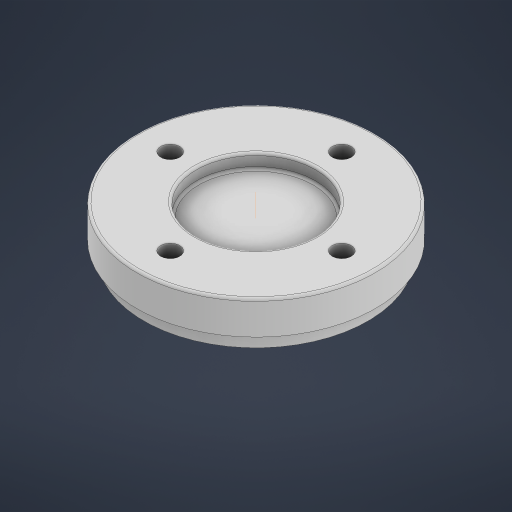
# Autodesk Inventor part: sf_Cylinder_Front_Lid_1
Saved by Autodesk Inventor 2024 (Build 280153000, 153)
## iProperties
Created: 2024-03-20
Part Number: sf_Cylinder_Front_Lid_1
Material: Generisch
Document SubType Name: Modeling
Designer: Simon
Density: 1 g/cm^3
Appearance: Vorgabe
Author: Simon
Autodesk Inventor part; units mm, degrees
ref_plane "YZ Plane" through (0, 0, 0) normal (1, 0, 0) x (0, 1, 0)
ref_plane "XZ Plane" through (0, 0, 0) normal (0, 1, 0) x (-1, 0, 0)
ref_plane "XY Plane" through (0, 0, 0) normal (0, 0, 1) x (1, 0, 0)
sketch "Skizze1" plane through (0, 0, 0) normal (1, 0, 0) x (0, 1, 0)
  line L0 (12.5, 3) -> (12.5, -3) construction
  line L1 (-12.5, -3) -> (-12.5, 3) construction
  line L2 (6, 26.2642) -> (6, -26.2642) construction
  line L3 (-6, -26.2642) -> (-6, 26.2642) construction
  line L4 (14, 26.2642) -> (14, -26.2642) construction
  line L5 (-14, -26.2642) -> (-14, 26.2642) construction
  line L6 (23.5, 26.2642) -> (23.5, -26.2642) construction
  line L7 (-23.5, -26.2642) -> (-23.5, 26.2642) construction
  line L8 (12.5, -3) -> (0, -3)
  line L9 (0, -3) -> (0, -8)
  line L10 (0, -8) -> (6, -8)
  line L11 (6, -8) -> (6, -13)
  line L12 (6, -13) -> (14, -13)
  line L13 (14, -13) -> (14, -10)
  line L14 (25, 26.2642) -> (25, -26.2642) construction
  line L15 (-25, -26.2642) -> (-25, 26.2642) construction
  line L16 (14, -10) -> (23.5, -10)
  line L17 (23.5, -10) -> (23.5, -7)
  line L18 (23.5, -7) -> (25, -7)
  line L19 (25, -7) -> (25, 0)
  line L20 (12.5, -3) -> (12.5, 0)
  line L21 (25, 0) -> (12.5, 0)
  point P0 (0, 0)
  dimension "d1" = 6
  dimension "d5" = 5
  dimension "d6" = 6
  dimension "d7" = 5
  dimension "d8" = 3
  dimension "d9" = 47
  dimension "d10" = 50
  dimension "d11" = 3
  constraints: 44 end point, 7 point on line, 5 parallel, 5 perpendicular, 2 midpoint, 1 horizontal
  measures "d1" distance of L0.start L0.end
  measures "d5" distance of L8.end L9.end
  measures "d6" distance of L9.end L10.end
  measures "d7" distance of L10.end L11.end
  measures "d8" distance of L12.end L13.end
  measures "d9" distance between parallel lines of L7 L6
  measures "d10" distance of L14.end L15.start
  measures "d11" distance of L16.end L17.end
revolve "Umdrehung1" add sketch "Skizze1" angle 360 about axis through (0, 0, -3) along (0, 0, -1)
sketch "Skizze2" plane through (0, 0, -10) normal (0, 0, -1) x (-1, 0, 0)
  circle A0 centre (0, 0) radius 18 construction
  circle A1 centre (0, 18) radius 2
  dimension "d13" = 36
  dimension "d14" = 4
  constraints: 1 centre point, 1 coincident, 1 vertical alignment, 2 other
  measures "d14" diameter of A1
extrude "Extrusion1" cut sketch "Skizze2" against normal up to surface (10 mm away)
pattern_circular "Runde Anordnung1" count 4 over 360 about axis through (0, 0, -10.5) along (0, 0, -1) of "Extrusion1"
sketch "Skizze3" plane through (0, 0, -13) normal (0, 0, -1) x (-1, 0, 0)
  line L0 (0, 0) -> (-21.5822, 21.5822) construction
  line L1 (0, 0) -> (30.5219, 0) construction
  line L2 (-16.2635, 9.1924) -> (-9.1924, 16.2635)
  line L3 (-9.1924, 16.2635) -> (-3.5355, 10.6066)
  line L4 (-3.5355, 10.6066) -> (-10.6066, 3.5355)
  line L5 (-10.6066, 3.5355) -> (-16.2635, 9.1924)
  circle A0 centre (0, 0) radius 14 projected
  line L6 (-16.2635, 9.1924) -> (-3.5355, 10.6066) construction
  line L7 (-9.1924, 16.2635) -> (-10.6066, 3.5355) construction
  point P0 (-9.8995, 9.8995)
  point P1 (-5.7111, 12.7822)
  point P2 (-12.7822, 5.7111)
  dimension "d20" = 135
  dimension "d21" = 10
  dimension "d22" = 8
  constraints: 16 end point, 2 midpoint, 2 parallel, 1 equal length, 1 horizontal, 1 perpendicular, 1 point on line, 2 other
  measures "d20" angle of L1 L0
  measures "d21" distance of L2.start L2.end
  measures "d22" distance of L2.end L3.end
extrude "Extrusion2" cut sketch "Skizze3" against normal up to surface (3 mm away) contours A0 L3 L4 L5 picked at (-7.5887, 8.3902)
fillet "Rundung1" radius 1.5 2 edges at (3.5355, 10.6066, -11.5) (10.6066, 3.5355, -11.5)
fillet "Rundung2" radius 0.5 3 edges at (0, -12.5, 0) (0, -12.5, -3) (0, -25, 0)
